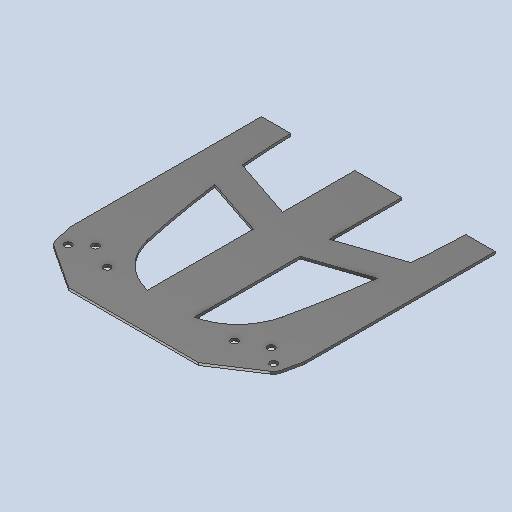
# Autodesk Inventor part: ABS Intake Hood
Saved by Autodesk Inventor 2025.1 (Build 291241020, 241B)
## iProperties
Created: 2024-12-30
Part Number: ABS Intake Hood
Material: Generic
Document SubType Name: Modeling
Designer: Juan
Density: 1 g/cm^3
Appearance: Default
Author: Juan
Autodesk Inventor part; units mm, degrees
ref_plane "YZ Plane" through (0, 0, 0) normal (1, 0, 0) x (0, 1, 0)
ref_plane "XZ Plane" through (0, 0, 0) normal (0, 1, 0) x (-1, 0, 0)
ref_plane "XY Plane" through (0, 0, 0) normal (0, 0, 1) x (1, 0, 0)
sketch "Sketch1" plane through (0, 0, 0) normal (0, 1, 0) x (-1, 0, 0)
  circle A0 centre (56.9406, -14.9623) radius 2.3241
  circle A1 centre (66.6693, -6.7989) radius 2.3241
  circle A2 centre (41.2693, -6.7989) radius 2.3241
  circle A3 centre (-41.6882, -6.7989) radius 2.3241
  circle A4 centre (-57.3594, -14.9623) radius 2.3241
  circle A5 centre (-67.0882, -6.7989) radius 2.3241
  arc A6 (-59.7156, -7.3708) -> (-58.0844, -7.6169) centre (-58.6976, -6.1526) ccw
  line L0 (-59.7156, -7.3708) -> (-85.288, 13.999)
  arc A7 (-43.7185, -2.4382) -> (-58.0844, -7.6169) centre (0.2546, -146.9346) ccw
  arc A8 (-43.7185, -2.4382) -> (-37.2086, 0.6056) centre (-51.1134, 21.8615) ccw
  arc A9 (-69.7478, -12.8722) -> (-69.4607, -10.2448) centre (-70.4786, -11.4629) ccw
  line L1 (-99.204, 14.6104) -> (-69.4607, -10.2448)
  arc A10 (-69.7478, -12.8722) -> (-78.2828, -17.6558) centre (-0.2094, -146.9516) ccw
  arc A11 (-16.3345, 6.2393) -> (-15.3068, 3.3313) centre (-15.4655, 4.9108) ccw
  arc A12 (14.8879, 3.3313) -> (-15.3068, 3.3313) centre (-0.2094, -146.9516) ccw
  arc A13 (14.8879, 3.3313) -> (15.9157, 6.2393) centre (15.0466, 4.9108) ccw
  arc A14 (37.2538, 0.5886) -> (43.7637, -2.4551) centre (51.1586, 21.8446) ccw
  arc A15 (58.1296, -7.6339) -> (43.7637, -2.4551) centre (-0.2094, -146.9516) ccw
  line L2 (85.3331, 13.982) -> (59.7607, -7.3877)
  arc A16 (58.1296, -7.6339) -> (59.7607, -7.3877) centre (58.7428, -6.1696) ccw
  line L3 (69.0418, -10.2448) -> (98.7851, 14.6104)
  arc A17 (69.0418, -10.2448) -> (69.3289, -12.8722) centre (70.0598, -11.4629) ccw
  arc A18 (77.8639, -17.6558) -> (69.3289, -12.8722) centre (-0.2094, -146.9516) ccw
  line L4 (66.6693, -6.7989) -> (41.2693, -6.7989)
  line L5 (0, 0) -> (0, 4.0875)
  circle A19 centre (66.6693, -6.7989) radius 3.9782
  circle A20 centre (41.2693, -6.7989) radius 4.9026
  line L6 (66.6693, -2.8207) -> (41.4483, -1.8996)
  circle A21 centre (56.9406, -14.9623) radius 4.1852
  line L7 (69.4813, -9.613) -> (60.0669, -17.7447)
  line L8 (54.6165, -18.4429) -> (39.1949, -11.241)
  line L9 (56.9406, -14.9623) -> (56.9406, -141.9623)
  arc A22 (56.9406, -141.9623) -> (36.3667, -6.7989) centre (-501.2889, -157.7854) ccw
  line L10 (56.9406, -141.9623) -> (75.9906, -141.9623)
  line L11 (75.9906, -141.9623) -> (75.9906, -17.7447)
  line L12 (75.9906, -17.7447) -> (65.708, -12.8722)
  circle A23 centre (-66.6693, -6.7989) radius 3.9782
  circle A24 centre (-41.2693, -6.7989) radius 4.9026
  line L13 (-66.6693, -2.8207) -> (-41.4483, -1.8996)
  circle A25 centre (-56.9406, -14.9623) radius 4.1852
  line L14 (-69.4813, -9.613) -> (-60.0669, -17.7447)
  arc A26 (-36.3667, -6.7989) -> (-56.9406, -141.9623) centre (501.2889, -157.7854) ccw
  line L15 (-56.9406, -141.9623) -> (-75.9906, -141.9623)
  line L16 (-75.9906, -141.9623) -> (-75.9906, -17.7447)
  line L17 (-75.9906, -17.7447) -> (-65.708, -12.8722)
  arc A27 (42.2115, -1.9275) -> (-42.2115, -1.9275) centre (0, -148.5156) ccw
  arc A28 (39.6774, -11.4417) -> (-39.7321, -11.4576) centre (0, -148.5156) ccw
  point P0 (-37.4811, -10.825)
  point P1 (37.4811, -10.825)
  dimension "d0" = 127
  dimension "d1" = 19.05
  constraints: 48 point on circle, 36 end point, 28 centre point, 13 symmetric about line, 6 tangent, 5 point on line, 3 coincident, 2 horizontal, 2 vertical, 1 perpendicular, 7 other
  measures "d0" distance of L9.start L9.end
  measures "d1" distance of L9.end L10.end
extrude "Extrusion1" add sketch "Sketch1" along normal blind 1.5875 contours L0 L13 A8 A7 A6 | A6 A7 A8 A24 A26 L15 L16 L17 L14 A23 L13 L0 | A23 L14 | L13 A24 A8 | A27 L6 A20 A22 A28 A26 A24 L13 | A24 A26 | A26 A24 | L6 L2 L4 A15 A14 | A14 A20 L6 | A14 A15 L4 A20 | A20 A22 | L6 A19 L2 | A28 L8 A21 L9 A22 | A22 A20 L8 A28 | L4 A15 A16 L2 A19 L7 A21 L8 A20 | A22 A20 | A19 L4 L2 | A19 L7 | L9 A21 L7 L12 L11 L10 | L4 L2 A16 A15 | A21 | A25 picked at (-63.4219, -7.1214) picked at (63.3048, -7.3068)
fillet "Fillet1" radius 38.1 2 edges at (37.4811, 0.7937, -10.825) (-37.4811, 0.7937, -10.825)
sketch "Sketch2" plane through (0, 1.5875, 0) normal (0, 1, 0) x (1, 0, 0)
  line L0 (0, 0) -> (0, -4.0291)
  arc A0 (-42.2115, 1.9275) -> (42.2115, 1.9275) centre (0, 148.5156) ccw projected
  line L1 (42.2115, 1.9275) -> (66.6693, 2.8207) projected
  arc A1 (66.6693, 2.8207) -> (69.4813, 9.613) centre (66.6693, 6.7989) ccw projected
  line L2 (69.4813, 9.613) -> (65.708, 12.8722) projected
  line L3 (65.708, 12.8722) -> (75.9906, 17.7447) projected
  line L4 (75.9906, 17.7447) -> (75.9906, 141.9623) projected
  line L5 (75.9906, 141.9623) -> (56.9406, 141.9623) projected
  arc A2 (43.6777, 35.794) -> (56.9406, 141.9623) centre (-501.2889, 157.7854) ccw projected
  arc A3 (8.8646, 6.0903) -> (43.6777, 35.794) centre (6.4979, 44.1168) ccw projected
  arc A4 (-8.8646, 6.0903) -> (8.8646, 6.0903) centre (0, 148.5156) ccw projected
  arc A5 (-43.6777, 35.794) -> (-8.8646, 6.0903) centre (-6.4979, 44.1168) ccw projected
  arc A6 (-56.9406, 141.9623) -> (-43.6777, 35.794) centre (501.2889, 157.7854) ccw projected
  line L6 (-56.9406, 141.9623) -> (-75.9906, 141.9623) projected
  line L7 (-75.9906, 141.9623) -> (-75.9906, 17.7447) projected
  line L8 (-75.9906, 17.7447) -> (-65.708, 12.8722) projected
  line L9 (-65.708, 12.8722) -> (-69.4813, 9.613) projected
  arc A7 (-69.4813, 9.613) -> (-66.6693, 2.8207) centre (-66.6693, 6.7989) ccw projected
  line L10 (-66.6693, 2.8207) -> (-42.2115, 1.9275) projected
  arc A8 (-42.2115, 1.9275) -> (42.2115, 1.9275) centre (0, 148.5156) ccw projected
  circle A9 centre (-41.2693, 6.7989) radius 2.3241 projected
  circle A10 centre (-66.6693, 6.7989) radius 2.3241 projected
  circle A11 centre (57.3594, 14.9623) radius 2.3241 projected
  circle A12 centre (67.0882, 6.7989) radius 2.3241 projected
  circle A13 centre (41.6882, 6.7989) radius 2.3241 projected
  circle A14 centre (-56.9406, 14.9623) radius 2.3241 projected
  circle A15 centre (67.0882, 6.7989) radius 6.35
  line L11 (73.2907, 5.4382) -> (75.9906, 17.7447)
  line L12 (42.2115, 1.9275) -> (66.7086, 0.4603)
  circle A16 centre (-67.0882, 6.7989) radius 6.35
  line L13 (-73.2907, 5.4382) -> (-75.9906, 17.7447)
  line L14 (-42.2115, 1.9275) -> (-66.7086, 0.4603)
  point P0 (-42.2115, 1.9275)
  dimension "d5" = 12.7
  constraints: 10 end point, 5 point on circle, 4 symmetric about line, 2 centre point, 2 tangent, 1 coincident, 1 vertical, 1 other
  measures "d5" diameter of A15
extrude "Extrusion2" add sketch "Sketch2" against normal blind 1.5875 contours L14 A16 L10 | A16 L8 L9 A7 L10 | L1 A15 L12 | L13 L8 A16 | L1 A1 L2 L3 A15 | L3 L11 A15 picked at (-67.6214, 11.869) picked at (67.6293, 11.8682)
sketch "Sketch3" plane through (0, 1.5875, 0) normal (0, 1, 0) x (1, 0, 0)
  line L0 (75.9906, 17.7447) -> (75.9906, 141.9623) projected
  line L1 (75.9906, 141.9623) -> (56.9406, 141.9623) projected
  arc A0 (43.6777, 35.794) -> (56.9406, 141.9623) centre (-501.2889, 157.7854) ccw projected
  arc A1 (8.8646, 6.0903) -> (43.6777, 35.794) centre (6.4979, 44.1168) ccw projected
  arc A2 (-8.8646, 6.0903) -> (8.8646, 6.0903) centre (0, 148.5156) ccw projected
  arc A3 (-43.6777, 35.794) -> (-8.8646, 6.0903) centre (-6.4979, 44.1168) ccw projected
  arc A4 (-56.9406, 141.9623) -> (-43.6777, 35.794) centre (501.2889, 157.7854) ccw projected
  line L2 (-56.9406, 141.9623) -> (-75.9906, 141.9623) projected
  line L3 (-75.9906, 141.9623) -> (-75.9906, 17.7447) projected
  line L4 (-75.9906, 17.7447) -> (-73.2907, 5.4382) projected
  arc A5 (-73.2907, 5.4382) -> (-66.7086, 0.4603) centre (-67.0882, 6.7989) ccw projected
  line L5 (-66.7086, 0.4603) -> (-42.2115, 1.9275) projected
  arc A6 (-42.2115, 1.9275) -> (42.2115, 1.9275) centre (0, 148.5156) ccw projected
  line L6 (42.2115, 1.9275) -> (66.7086, 0.4603) projected
  arc A7 (66.7086, 0.4603) -> (73.2907, 5.4382) centre (67.0882, 6.7989) ccw projected
  line L7 (73.2907, 5.4382) -> (75.9906, 17.7447) projected
  circle A8 centre (-41.2693, 6.7989) radius 2.3241 projected
  circle A9 centre (-66.6693, 6.7989) radius 2.3241 projected
  circle A10 centre (57.3594, 14.9623) radius 2.3241 projected
  circle A11 centre (67.0882, 6.7989) radius 2.3241 projected
  circle A12 centre (41.6882, 6.7989) radius 2.3241 projected
  circle A13 centre (-56.9406, 14.9623) radius 2.3241 projected
  line L8 (-75.9906, 141.9623) -> (-75.9906, 17.7447) projected
  line L9 (75.9906, 17.7447) -> (-75.9906, 17.7447)
  line L10 (-75.9906, 17.7447) -> (0, 17.7447)
  line L11 (0, 17.7447) -> (0, 5.8147)
  arc A14 (-8.8646, 6.0903) -> (8.8646, 6.0903) centre (0, 148.5156) ccw projected
  line L12 (8.8646, 141.9623) -> (-8.8646, 141.9623)
  line L13 (8.8646, 141.9623) -> (15.2146, 141.9623)
  line L14 (-8.8646, 141.9623) -> (-15.2146, 141.9623)
  line L15 (-15.2146, 141.9623) -> (-15.2146, 7.0273)
  line L16 (15.2146, 141.9623) -> (15.2146, 7.0273)
  point P0 (0, 0)
  dimension "d8" = 6.35
  dimension "d9" = 6.35
  constraints: 16 end point, 3 point on circle, 2 horizontal, 2 perpendicular, 1 midpoint, 1 parallel
  measures "d8" distance of L12.start L13.end
  measures "d9" distance of L12.end L14.end
extrude "Extrusion3" add sketch "Sketch3" against normal blind 1.5875 contours A1 A2 L11 L9 L16 | L9 L15 L14 L12 L13 L16 | L11 A2 A3 L15 L9
sketch "Sketch4" plane through (0, 1.5875, 0) normal (0, 1, 0) x (1, 0, 0)
  line L0 (75.9906, 17.7447) -> (75.9906, 141.9623) projected
  line L1 (75.9906, 141.9623) -> (56.9406, 141.9623) projected
  arc A0 (43.6777, 35.794) -> (56.9406, 141.9623) centre (-501.2889, 157.7854) ccw projected
  arc A1 (15.2146, 7.0273) -> (43.6777, 35.794) centre (6.4979, 44.1168) ccw projected
  line L2 (15.2146, 7.0273) -> (15.2146, 141.9623) projected
  line L3 (15.2146, 141.9623) -> (-15.2146, 141.9623) projected
  line L4 (-15.2146, 141.9623) -> (-15.2146, 7.0273) projected
  arc A2 (-43.6777, 35.794) -> (-15.2146, 7.0273) centre (-6.4979, 44.1168) ccw projected
  arc A3 (-56.9406, 141.9623) -> (-43.6777, 35.794) centre (501.2889, 157.7854) ccw projected
  line L5 (-56.9406, 141.9623) -> (-75.9906, 141.9623) projected
  line L6 (-75.9906, 141.9623) -> (-75.9906, 17.7447) projected
  line L7 (-75.9906, 17.7447) -> (-73.2907, 5.4382) projected
  arc A4 (-73.2907, 5.4382) -> (-66.7086, 0.4603) centre (-67.0882, 6.7989) ccw projected
  line L8 (-66.7086, 0.4603) -> (-42.2115, 1.9275) projected
  arc A5 (-42.2115, 1.9275) -> (42.2115, 1.9275) centre (0, 148.5156) ccw projected
  line L9 (42.2115, 1.9275) -> (66.7086, 0.4603) projected
  arc A6 (66.7086, 0.4603) -> (73.2907, 5.4382) centre (67.0882, 6.7989) ccw projected
  line L10 (73.2907, 5.4382) -> (75.9906, 17.7447) projected
  circle A7 centre (-41.2693, 6.7989) radius 2.3241 projected
  circle A8 centre (-66.6693, 6.7989) radius 2.3241 projected
  circle A9 centre (57.3594, 14.9623) radius 2.3241 projected
  circle A10 centre (67.0882, 6.7989) radius 2.3241 projected
  circle A11 centre (41.6882, 6.7989) radius 2.3241 projected
  circle A12 centre (-56.9406, 14.9623) radius 2.3241 projected
  line L11 (-15.2146, 44.1168) -> (15.2146, 44.1168)
  line L12 (15.2146, 44.1168) -> (15.2146, 75.8668)
  line L13 (15.2146, 75.8668) -> (52.8576, 88.5598)
  arc A13 (43.6777, 35.794) -> (56.9406, 141.9623) centre (-501.2889, 157.7854) ccw projected
  line L14 (15.2146, 75.8668) -> (15.2146, 94.9168)
  line L15 (15.2146, 141.9623) -> (15.2146, 7.0273) projected
  line L16 (15.2146, 94.9168) -> (54.9699, 108.3221)
  line L17 (0, 44.1168) -> (0, 50.0619)
  line L18 (-15.2146, 75.8668) -> (-52.8576, 88.5598)
  line L19 (-15.2146, 94.9168) -> (-54.9699, 108.3221)
  point P0 (0, 0)
  dimension "d12" = 31.75
  dimension "d13" = 19.05
  constraints: 16 end point, 4 point on line, 4 symmetric about line, 2 point on circle, 1 midpoint, 1 parallel, 1 perpendicular, 1 vertical
  measures "d12" distance of L11.end L12.end
  measures "d13" distance of L12.end L14.end
extrude "Extrusion4" add sketch "Sketch4" against normal blind 1.5875 contours A0 L13 L2 L16 | L4 L18 A3 L19
sketch "Sketch5" plane through (0, 1.5875, 0) normal (0, 1, 0) x (1, 0, 0)
  arc A0 (43.6777, 35.794) -> (52.8576, 88.5598) centre (-501.2889, 157.7854) ccw projected
  arc A1 (15.2146, 7.0273) -> (43.6777, 35.794) centre (6.4979, 44.1168) ccw projected
  line L0 (15.2146, 7.0273) -> (15.2146, 75.8668) projected
  line L1 (15.2146, 75.8668) -> (52.8576, 88.5598) projected
  line L2 (54.9699, 108.3221) -> (15.2146, 94.9168) projected
  line L3 (15.2146, 94.9168) -> (15.2146, 141.9623) projected
  line L4 (15.2146, 141.9623) -> (-15.2146, 141.9623) projected
  line L5 (-15.2146, 141.9623) -> (-15.2146, 94.9168) projected
  line L6 (-15.2146, 94.9168) -> (-54.9699, 108.3221) projected
  arc A2 (-56.9406, 141.9623) -> (-54.9699, 108.3221) centre (501.2889, 157.7854) ccw projected
  line L7 (-56.9406, 141.9623) -> (-75.9906, 141.9623) projected
  line L8 (-75.9906, 141.9623) -> (-75.9906, 17.7447) projected
  line L9 (-75.9906, 17.7447) -> (-73.2907, 5.4382) projected
  arc A3 (-73.2907, 5.4382) -> (-66.7086, 0.4603) centre (-67.0882, 6.7989) ccw projected
  line L10 (-66.7086, 0.4603) -> (-42.2115, 1.9275) projected
  arc A4 (-42.2115, 1.9275) -> (42.2115, 1.9275) centre (0, 148.5156) ccw projected
  line L11 (42.2115, 1.9275) -> (66.7086, 0.4603) projected
  arc A5 (66.7086, 0.4603) -> (73.2907, 5.4382) centre (67.0882, 6.7989) ccw projected
  line L12 (73.2907, 5.4382) -> (75.9906, 17.7447) projected
  line L13 (75.9906, 17.7447) -> (75.9906, 141.9623) projected
  line L14 (75.9906, 141.9623) -> (56.9406, 141.9623) projected
  arc A6 (54.9699, 108.3221) -> (56.9406, 141.9623) centre (-501.2889, 157.7854) ccw projected
  line L15 (-52.8576, 88.5598) -> (-15.2146, 75.8668) projected
  line L16 (-15.2146, 75.8668) -> (-15.2146, 7.0273) projected
  arc A7 (-43.6777, 35.794) -> (-15.2146, 7.0273) centre (-6.4979, 44.1168) ccw projected
  arc A8 (-52.8576, 88.5598) -> (-43.6777, 35.794) centre (501.2889, 157.7854) ccw projected
  circle A9 centre (-41.2693, 6.7989) radius 2.3241 projected
  circle A10 centre (-66.6693, 6.7989) radius 2.3241 projected
  circle A11 centre (57.3594, 14.9623) radius 2.3241 projected
  circle A12 centre (67.0882, 6.7989) radius 2.3241 projected
  circle A13 centre (41.6882, 6.7989) radius 2.3241 projected
  circle A14 centre (-56.9406, 14.9623) radius 2.3241 projected
  line L17 (-42.2115, 1.9275) -> (-42.2115, -17.1225)
  line L18 (-70.5723, 1.4901) -> (-42.2115, -17.1225)
  line L19 (0, 0) -> (0, -4.0291)
  arc A15 (-73.2907, 5.4382) -> (-66.7086, 0.4603) centre (-67.0882, 6.7989) ccw projected
  line L20 (42.2115, 1.9275) -> (42.2115, -17.1225)
  line L21 (70.5723, 1.4901) -> (42.2115, -17.1225)
  line L22 (-42.2115, -17.1225) -> (42.2115, -17.1225)
  dimension "d16" = 19.05
  constraints: 12 end point, 2 point on circle, 2 symmetric about line, 1 perpendicular, 1 tangent, 1 vertical
  measures "d16" distance of L10.end L17.end
extrude "Extrusion5" add sketch "Sketch5" against normal blind 1.5875 contours L21 L20 L11 A5 | L22 L17 A4 L20 | L18 A3 L10 L17
body "Solid1"
